Trimix_Enclosure_A2 (Autodesk Fusion 360 design; units mm, degrees)
description: designed concept
description: Owner measured 116.8x69.3x13.7; casing retained, factory back removed; interior drawing-derived
description: Drawing-derived visual reconstruction; connector positions and factory mounting holes require confirmation
description: nominal generic hardware; not supplier-authenticated CAD
part number: GEN-M3-BHCS-L8-AF2
part number: GEN-M3-HEATSET-OD4.2-L5
description: Owner-measured occupied FMA FPML1S2P050C envelope 42 W x 80.4 H x 20.35 D mm; pocket and local frame details provisional
description: Owner capacity 3400 mAh; 18.2 mm diameter x 69 mm cylinder is a dimensional visual reference, not measured cell CAD
description: RCY/BEC-style red two-wire battery disconnect retained by owner; provisional 12 x 10 x 4 mm reference body, not selected manufacturer CAD
description: RCY/BEC-style red disconnect mating reference; provisional 12 x 10 x 2.2 mm, not selected manufacturer CAD
description: 2 mm printed carrier; future PCB and disconnect notches, procurement pending
description: Space allocation only; no claim that the charging and sensor circuitry is routed or fitted
part number: GEN-M2-SHCS-L7-AF1.5
part number: GEN-M2-HEATSET-OD3.2-L4
description: Rear-release concept. Factory frame capture lip, pad contact and preload require measurement; not a validated display fastening detail
part number: GEN-M2-SHCS-L5-AF1.5
description: 12 mm purchased button; barrel, nut and terminals are conservative unmeasured references
description: Designed metal faceplate reference: 2.3 mm bulk, locally 1.80 mm; material/process and sealing unqualified; not a printed-wall exception
description: Designed removable printed support with >=2 mm nominal flange and boss walls; housing retention and physical fit unqualified
description: Provisional 13.6 x 16 x 0.60 mm board; connector straddle relief and mounting references only; no final circuit layout
description: GCT USB4720 Rev B drawing-derived reconstruction; manufacturer STEP download blocked. Simplified shell, tongue and gasket; not exact supplier CAD.
part number: USB4720-03-A-DRAWING-REFERENCE
description: GCT USB4720 Rev B drawing-derived reconstruction; manufacturer STEP download blocked. Simplified shell, tongue and gasket; not exact supplier CAD. Gasket is an uncompressed visual clearance reference, not seal simulation.
description: Illustrative contact stripes; not electrical pin geometry or PCB footprint
part number: GEN-M2-SHCS-L4-AF1.5
part number: GEN-M2-SHCS-L6-AF1.5
description: Designed printed L-clamp; 2 mm strap/stalk, 0.2 mm lateral stop clearance; physical fit and hand access pending
description: Separate 2 mm internal lid; gasket and seal groove deferred
description: Datasheet dimensional envelope: body Ø29.3x31.75, neck Ø16x6.5; no exact threads or supplier CAD
description: Unmeasured 6.5x10x10 connector and wire clearance
description: Drawing-derived PCB thickness1.6, can Ø20x16.7, opposite3.45 mm header allowance. Header profile and finishes illustrative; original total envelope remains reserved.
description: Full19x9.5x14 body rotated to X9.5,Y14,Z19; no manufacturer CAD available
description: Conservative clearance block for full26±1 mm leads, +Y orientation; not a physical solid lead bundle
description: Provisional12x17x5 GYBMEP envelope retained. Board thickness, pad holes, cap, IC placement and finishes are illustrative; module identity and all mounting dimensions remain unverified.
description: Nominal8 mm OD/5 mm ID straight fitting reference; actual part, flange, seal and hose bend unmeasured
description: Nominal4.4 mm OD feedthrough reference; wire potting, actual gland, cable diameter and bends unverified
description: Designed concept; nominal 2 mm walls; seal geometry and pressure qualification deferred
Autodesk Fusion 360 part; units mm, degrees
(part 1 of 6)
ref_plane "WorkPlane1" through (0, 0, 0) normal (0, 0, 1) x (1, 0, 0) in component "01 Tapered printed housing"
sketch "Front silhouette" plane through (0, 0, 0) normal (0, 0, 1) x (1, 0, 0) in component "01 Tapered printed housing"
  line L0 (0, 0) -> (75, 0)
  line L1 (75, 0) -> (75, 125)
  line L2 (75, 125) -> (0, 125)
  line L3 (0, 125) -> (0, 0)
  dimension "d45" = 75
  dimension "d46" = 125
  constraint horizontal L0
  constraint vertical L1
  constraint horizontal L2
  constraint vertical L3
  measures "d45" horizontal distance of L0.start L0.end
  measures "d46" vertical distance of L0.end L1.end
ref_plane "WorkPlane2" through (0, 0, 53.6) normal (0, 0, 1) x (1, 0, 0) in component "01 Tapered printed housing"
sketch "Rear silhouette" plane through (0, 0, 53.6) normal (0, 0, 1) x (1, 0, 0) in component "01 Tapered printed housing"
  line L0 (0.25, 0.25) -> (74.75, 0.25)
  line L1 (74.75, 0.25) -> (74.75, 124.75)
  line L2 (74.75, 124.75) -> (0.25, 124.75)
  line L3 (0.25, 124.75) -> (0.25, 0.25)
  dimension "d49" = 0.25
  dimension "d50" = 0.25
  dimension "d51" = 74.5
  dimension "d52" = 124.5
  constraint horizontal L0
  constraint vertical L1
  constraint horizontal L2
  constraint vertical L3
  measures "d49" horizontal distance of origin L0.start
  measures "d50" vertical distance of origin L0.start
  measures "d51" horizontal distance of L0.start L0.end
  measures "d52" vertical distance of L0.end L1.end
loft "Gentle rearward taper" add profiles "Front silhouette", "Rear silhouette" section 1 section 2 makes body 1 in component "01 Tapered printed housing"
fillet "Soft housing corners" radius 6 4 edges at (0.125, 0.125, 26.8) (0.125, 124.875, 26.8) (74.875, 0.125, 26.8) (74.875, 124.875, 26.8) on bodies 1 in component "01 Tapered printed housing"
ref_plane "WorkPlane3" through (0, 0, 14.5) normal (0, 0, 1) x (1, 0, 0) in component "01 Tapered printed housing"
sketch "Rear service cavity sketch" plane through (0, 0, 14.5) normal (0, 0, 1) x (1, 0, 0) in component "01 Tapered printed housing"
  line L0 (2.4, 2.4) -> (72.6, 2.4)
  line L1 (72.6, 2.4) -> (72.6, 122.6)
  line L2 (72.6, 122.6) -> (2.4, 122.6)
  line L3 (2.4, 122.6) -> (2.4, 2.4)
  dimension "d57" = 2.4
  dimension "d58" = 2.4
  dimension "d59" = 70.2
  dimension "d60" = 120.2
  constraint horizontal L0
  constraint vertical L1
  constraint horizontal L2
  constraint vertical L3
  measures "d57" horizontal distance of origin L0.start
  measures "d58" vertical distance of origin L0.start
  measures "d59" horizontal distance of L0.start L0.end
  measures "d60" vertical distance of L0.end L1.end
extrude "Rear service cavity" cut sketch "Rear service cavity sketch" along normal blind 56 bodies 1 in component "01 Tapered printed housing"
fillet "Inside cavity corner rounds" radius 3.6 4 edges at (72.6, 2.4, 34.05) (2.4, 2.4, 34.05) (2.4, 122.6, 34.05) (72.6, 122.6, 34.05) on bodies 1 in component "01 Tapered printed housing"
ref_plane "WorkPlane4" through (0, 0, -1) normal (0, 0, 1) x (1, 0, 0) in component "01 Tapered printed housing"
sketch "Front-removable factory display opening sketch" plane through (0, 0, -1) normal (0, 0, 1) x (1, 0, 0) in component "01 Tapered printed housing"
  line L0 (2.45, 3.7) -> (72.55, 3.7)
  line L1 (72.55, 3.7) -> (72.55, 121.3)
  line L2 (72.55, 121.3) -> (2.45, 121.3)
  line L3 (2.45, 121.3) -> (2.45, 3.7)
  dimension "d67" = 2.45
  dimension "d68" = 3.7
  dimension "d69" = 70.1
  dimension "d70" = 117.6
  constraint horizontal L0
  constraint vertical L1
  constraint horizontal L2
  constraint vertical L3
  measures "d67" horizontal distance of origin L0.start
  measures "d68" vertical distance of origin L0.start
  measures "d69" horizontal distance of L0.start L0.end
  measures "d70" vertical distance of L0.end L1.end
extrude "Front-removable factory display opening" cut sketch "Front-removable factory display opening sketch" along normal blind 16 bodies 1 in component "01 Tapered printed housing"
ref_plane "WorkPlane5" through (-1, 0, 0) normal (1, 0, 0) x (0, 1, 0) in component "01 Tapered printed housing"
sketch "Gas fitting wall passages sketch" plane through (-1, 0, 0) normal (1, 0, 0) x (0, 0, -1) in component "01 Tapered printed housing"
  circle A0 centre (-23, 105) radius 4.5
  dimension "d76" = 105
  dimension "d77" = 4.5
  measures "d76" vertical distance of origin A0.centre
  measures "d77" radius of A0
extrude "Gas fitting wall passages" cut sketch "Gas fitting wall passages sketch" along normal blind 77 bodies 1 in component "01 Tapered printed housing"
ref_plane "WorkPlane6" through (-1, 0, 0) normal (1, 0, 0) x (0, 1, 0) in component "01 Tapered printed housing"
sketch "Right button panel opening sketch" plane through (-1, 0, 0) normal (1, 0, 0) x (0, 0, -1) in component "01 Tapered printed housing"
  circle A0 centre (-44.5, 45) radius 6
  dimension "d83" = 45
  dimension "d84" = 6
  measures "d83" vertical distance of origin A0.centre
  measures "d84" radius of A0
extrude "Right button panel opening" cut sketch "Right button panel opening sketch" along normal blind 4.4 bodies 1 in component "01 Tapered printed housing"
ref_plane "WorkPlane7" through (71.6, 0, 0) normal (1, 0, 0) x (0, 1, 0) in component "01 Tapered printed housing"
sketch "Left USB insert opening sketch" plane through (71.6, 0, 0) normal (1, 0, 0) x (0, 0, -1) in component "01 Tapered printed housing"
  line L0 (-35, 6) -> (-19, 6)
  line L1 (-19, 6) -> (-19, 26)
  line L2 (-19, 26) -> (-35, 26)
  line L3 (-35, 26) -> (-35, 6)
  dimension "d89" = 35
  dimension "d90" = 6
  dimension "d91" = 16
  dimension "d92" = 20
  constraint horizontal L0
  constraint vertical L1
  constraint horizontal L2
  constraint vertical L3
  measures "d89" horizontal distance of origin L0.start
  measures "d90" vertical distance of origin L0.start
  measures "d91" horizontal distance of L0.start L0.end
  measures "d92" vertical distance of L0.end L1.end
extrude "Left USB insert opening" cut sketch "Left USB insert opening sketch" along normal blind 4.4 bodies 1 in component "01 Tapered printed housing"
ref_plane "WorkPlane1" through (0, 0, 53.8) normal (0, 0, 1) x (1, 0, 0) in component "02 Single rear cover"
sketch "Single screw-fastened rear cover sketch" plane through (0, 0, 53.8) normal (0, 0, 1) x (1, 0, 0) in component "02 Single rear cover"
  line L0 (0.25, 0.25) -> (74.75, 0.25)
  line L1 (74.75, 0.25) -> (74.75, 124.75)
  line L2 (74.75, 124.75) -> (0.25, 124.75)
  line L3 (0.25, 124.75) -> (0.25, 0.25)
  dimension "d97" = 0.25
  dimension "d98" = 0.25
  dimension "d99" = 74.5
  dimension "d100" = 124.5
  constraint horizontal L0
  constraint vertical L1
  constraint horizontal L2
  constraint vertical L3
  measures "d97" horizontal distance of origin L0.start
  measures "d98" vertical distance of origin L0.start
  measures "d99" horizontal distance of L0.start L0.end
  measures "d100" vertical distance of L0.end L1.end
extrude "Single screw-fastened rear cover" add sketch "Single screw-fastened rear cover sketch" along normal blind 2.2 separate body makes body 2 in component "02 Single rear cover"
fillet "Rear cover corner rounds" radius 6 4 edges at (0.25, 124.75, 54.9) (74.75, 124.75, 54.9) (74.75, 0.25, 54.9) (0.25, 0.25, 54.9) on bodies 2 in component "02 Single rear cover"
ref_plane "WorkPlane1" through (0, 0, 0.4) normal (0, 0, 1) x (1, 0, 0) in component "03 Guition factory casing — measured envelope"
sketch "Guition retained factory frame sketch" plane through (0, 0, 0.4) normal (0, 0, 1) x (1, 0, 0) in component "03 Guition factory casing — measured envelope"
  line L0 (2.85, 4.1) -> (72.15, 4.1)
  line L1 (72.15, 4.1) -> (72.15, 120.9)
  line L2 (72.15, 120.9) -> (2.85, 120.9)
  line L3 (2.85, 120.9) -> (2.85, 4.1)
  dimension "d107" = 2.85
  dimension "d108" = 4.1
  dimension "d109" = 69.3
  dimension "d110" = 116.8
  constraint horizontal L0
  constraint vertical L1
  constraint horizontal L2
  constraint vertical L3
  measures "d107" horizontal distance of origin L0.start
  measures "d108" vertical distance of origin L0.start
  measures "d109" horizontal distance of L0.start L0.end
  measures "d110" vertical distance of L0.end L1.end
extrude "Guition retained factory frame" add sketch "Guition retained factory frame sketch" along normal blind 13.7 separate body makes body 3 in component "03 Guition factory casing — measured envelope"
fillet "Factory frame corner reference" radius 2 4 edges at (2.85, 120.9, 7.25) (72.15, 120.9, 7.25) (72.15, 4.1, 7.25) (2.85, 4.1, 7.25) on bodies 3 in component "03 Guition factory casing — measured envelope"
ref_plane "WorkPlane2" through (0, 0, 3.4) normal (0, 0, 1) x (1, 0, 0) in component "03 Guition factory casing — measured envelope"
sketch "Factory open rear cavity sketch" plane through (0, 0, 3.4) normal (0, 0, 1) x (1, 0, 0) in component "03 Guition factory casing — measured envelope"
  line L0 (4.8, 8.5) -> (70.2, 8.5)
  line L1 (70.2, 8.5) -> (70.2, 116.5)
  line L2 (70.2, 116.5) -> (4.8, 116.5)
  line L3 (4.8, 116.5) -> (4.8, 8.5)
  dimension "d117" = 4.8
  dimension "d118" = 8.5
  dimension "d119" = 65.4
  dimension "d120" = 108
  constraint horizontal L0
  constraint vertical L1
  constraint horizontal L2
  constraint vertical L3
  measures "d117" horizontal distance of origin L0.start
  measures "d118" vertical distance of origin L0.start
  measures "d119" horizontal distance of L0.start L0.end
  measures "d120" vertical distance of L0.end L1.end
extrude "Factory open rear cavity" cut sketch "Factory open rear cavity sketch" along normal blind 12 bodies 3 in component "03 Guition factory casing — measured envelope"
ref_plane "WorkPlane3" through (0, 0, 0.3) normal (0, 0, 1) x (1, 0, 0) in component "03 Guition factory casing — measured envelope"
sketch "Factory glass recess sketch" plane through (0, 0, 0.3) normal (0, 0, 1) x (1, 0, 0) in component "03 Guition factory casing — measured envelope"
  line L0 (4.1, 5.3) -> (70.9, 5.3)
  line L1 (70.9, 5.3) -> (70.9, 119.7)
  line L2 (70.9, 119.7) -> (4.1, 119.7)
  line L3 (4.1, 119.7) -> (4.1, 5.3)
  dimension "d125" = 4.1
  dimension "d126" = 5.3
  dimension "d127" = 66.8
  dimension "d128" = 114.4
  constraint horizontal L0
  constraint vertical L1
  constraint horizontal L2
  constraint vertical L3
  measures "d125" horizontal distance of origin L0.start
  measures "d126" vertical distance of origin L0.start
  measures "d127" horizontal distance of L0.start L0.end
  measures "d128" vertical distance of L0.end L1.end
extrude "Factory glass recess" cut sketch "Factory glass recess sketch" along normal blind 1.3 bodies 3 in component "03 Guition factory casing — measured envelope"
ref_plane "WorkPlane1" through (0, 0, 0.4) normal (0, 0, 1) x (1, 0, 0) in component "04 Guition front glass — drawing reference"
sketch "Black border glass sketch" plane through (0, 0, 0.4) normal (0, 0, 1) x (1, 0, 0) in component "04 Guition front glass — drawing reference"
  line L0 (4.1, 5.3) -> (70.9, 5.3)
  line L1 (70.9, 5.3) -> (70.9, 119.7)
  line L2 (70.9, 119.7) -> (4.1, 119.7)
  line L3 (4.1, 119.7) -> (4.1, 5.3)
  dimension "d133" = 4.1
  dimension "d134" = 5.3
  dimension "d135" = 66.8
  dimension "d136" = 114.4
  constraint horizontal L0
  constraint vertical L1
  constraint horizontal L2
  constraint vertical L3
  measures "d133" horizontal distance of origin L0.start
  measures "d134" vertical distance of origin L0.start
  measures "d135" horizontal distance of L0.start L0.end
  measures "d136" vertical distance of L0.end L1.end
extrude "Black border glass" add sketch "Black border glass sketch" along normal blind 1.2 separate body makes body 4 in component "04 Guition front glass — drawing reference"
ref_plane "WorkPlane2" through (0, 0, 0.3) normal (0, 0, 1) x (1, 0, 0) in component "04 Guition front glass — drawing reference"
sketch "Active face recess sketch" plane through (0, 0, 0.3) normal (0, 0, 1) x (1, 0, 0) in component "04 Guition front glass — drawing reference"
  line L0 (9.42, 15.7) -> (65.58, 15.7)
  line L1 (65.58, 15.7) -> (65.58, 109.3)
  line L2 (65.58, 109.3) -> (9.42, 109.3)
  line L3 (9.42, 109.3) -> (9.42, 15.7)
  dimension "d141" = 9.42
  dimension "d142" = 15.7
  dimension "d143" = 56.16
  dimension "d144" = 93.6
  constraint horizontal L0
  constraint vertical L1
  constraint horizontal L2
  constraint vertical L3
  measures "d141" horizontal distance of origin L0.start
  measures "d142" vertical distance of origin L0.start
  measures "d143" horizontal distance of L0.start L0.end
  measures "d144" vertical distance of L0.end L1.end
extrude "Active face recess" cut sketch "Active face recess sketch" along normal blind 0.2 bodies 4 in component "04 Guition front glass — drawing reference"
ref_plane "WorkPlane1" through (0, 0, 0.4) normal (0, 0, 1) x (1, 0, 0) in component "05 Active 4.3 inch screen"
sketch "480x800 active area sketch" plane through (0, 0, 0.4) normal (0, 0, 1) x (1, 0, 0) in component "05 Active 4.3 inch screen"
  line L0 (9.42, 15.7) -> (65.58, 15.7)
  line L1 (65.58, 15.7) -> (65.58, 109.3)
  line L2 (65.58, 109.3) -> (9.42, 109.3)
  line L3 (9.42, 109.3) -> (9.42, 15.7)
  dimension "d149" = 9.42
  dimension "d150" = 15.7
  dimension "d151" = 56.16
  dimension "d152" = 93.6
  constraint horizontal L0
  constraint vertical L1
  constraint horizontal L2
  constraint vertical L3
  measures "d149" horizontal distance of origin L0.start
  measures "d150" vertical distance of origin L0.start
  measures "d151" horizontal distance of L0.start L0.end
  measures "d152" vertical distance of L0.end L1.end
extrude "480x800 active area" add sketch "480x800 active area sketch" along normal blind 0.1 separate body makes body 5 in component "05 Active 4.3 inch screen"
ref_plane "WorkPlane1" through (0, 0, 8) normal (0, 0, 1) x (1, 0, 0) in component "06 Guition PCB and connectors — illustrative detail"
sketch "Guition PCB outline reference sketch" plane through (0, 0, 8) normal (0, 0, 1) x (1, 0, 0) in component "06 Guition PCB and connectors — illustrative detail"
  line L0 (4.97, 8.5) -> (70.03, 8.5)
  line L1 (70.03, 8.5) -> (70.03, 116.5)
  line L2 (70.03, 116.5) -> (4.97, 116.5)
  line L3 (4.97, 116.5) -> (4.97, 8.5)
  dimension "d157" = 4.97
  dimension "d158" = 8.5
  dimension "d159" = 65.06
  dimension "d160" = 108
  constraint horizontal L0
  constraint vertical L1
  constraint horizontal L2
  constraint vertical L3
  measures "d157" horizontal distance of origin L0.start
  measures "d158" vertical distance of origin L0.start
  measures "d159" horizontal distance of L0.start L0.end
  measures "d160" vertical distance of L0.end L1.end
extrude "Guition PCB outline reference" add sketch "Guition PCB outline reference sketch" along normal blind 1.6 separate body makes body 6 in component "06 Guition PCB and connectors — illustrative detail"
ref_plane "WorkPlane2" through (0, 0, 7.9) normal (0, 0, 1) x (1, 0, 0) in component "06 Guition PCB and connectors — illustrative detail"
sketch "Factory mounting clearance reference sketch" plane through (0, 0, 7.9) normal (0, 0, 1) x (1, 0, 0) in component "06 Guition PCB and connectors — illustrative detail"
  circle A0 centre (7.5, 11.2) radius 2.5
  dimension "d165" = 7.5
  dimension "d166" = 11.2
  dimension "d167" = 2.5
  measures "d165" horizontal distance of origin A0.centre
  measures "d166" vertical distance of origin A0.centre
  measures "d167" radius of A0
extrude "Factory mounting clearance reference" cut sketch "Factory mounting clearance reference sketch" along normal blind 1.8 bodies 6 in component "06 Guition PCB and connectors — illustrative detail"
ref_plane "WorkPlane3" through (0, 0, 7.9) normal (0, 0, 1) x (1, 0, 0) in component "06 Guition PCB and connectors — illustrative detail"
sketch "Factory mounting clearance reference sketch (1)" plane through (0, 0, 7.9) normal (0, 0, 1) x (1, 0, 0) in component "06 Guition PCB and connectors — illustrative detail"
  circle A0 centre (7.5, 113.8) radius 2.5
  dimension "d172" = 7.5
  dimension "d173" = 113.8
  dimension "d174" = 2.5
  measures "d172" horizontal distance of origin A0.centre
  measures "d173" vertical distance of origin A0.centre
  measures "d174" radius of A0
extrude "Factory mounting clearance reference (1)" cut sketch "Factory mounting clearance reference sketch (1)" along normal blind 1.8 bodies 6 in component "06 Guition PCB and connectors — illustrative detail"
ref_plane "WorkPlane4" through (0, 0, 7.9) normal (0, 0, 1) x (1, 0, 0) in component "06 Guition PCB and connectors — illustrative detail"
sketch "Factory mounting clearance reference sketch (2)" plane through (0, 0, 7.9) normal (0, 0, 1) x (1, 0, 0) in component "06 Guition PCB and connectors — illustrative detail"
  circle A0 centre (67.5, 11.2) radius 2.5
  dimension "d179" = 67.5
  dimension "d180" = 11.2
  dimension "d181" = 2.5
  measures "d179" horizontal distance of origin A0.centre
  measures "d180" vertical distance of origin A0.centre
  measures "d181" radius of A0
extrude "Factory mounting clearance reference (2)" cut sketch "Factory mounting clearance reference sketch (2)" along normal blind 1.8 bodies 6 in component "06 Guition PCB and connectors — illustrative detail"
ref_plane "WorkPlane5" through (0, 0, 7.9) normal (0, 0, 1) x (1, 0, 0) in component "06 Guition PCB and connectors — illustrative detail"
sketch "Factory mounting clearance reference sketch (3)" plane through (0, 0, 7.9) normal (0, 0, 1) x (1, 0, 0) in component "06 Guition PCB and connectors — illustrative detail"
  circle A0 centre (67.5, 113.8) radius 2.5
  dimension "d186" = 67.5
  dimension "d187" = 113.8
  dimension "d188" = 2.5
  measures "d186" horizontal distance of origin A0.centre
  measures "d187" vertical distance of origin A0.centre
  measures "d188" radius of A0
extrude "Factory mounting clearance reference (3)" cut sketch "Factory mounting clearance reference sketch (3)" along normal blind 1.8 bodies 6 in component "06 Guition PCB and connectors — illustrative detail"
ref_plane "WorkPlane6" through (0, 0, 9.6) normal (0, 0, 1) x (1, 0, 0) in component "06 Guition PCB and connectors — illustrative detail"
sketch "ESP32-P4 visual reference sketch" plane through (0, 0, 9.6) normal (0, 0, 1) x (1, 0, 0) in component "06 Guition PCB and connectors — illustrative detail"
  line L0 (15, 75) -> (31, 75)
  line L1 (31, 75) -> (31, 91)
  line L2 (31, 91) -> (15, 91)
  line L3 (15, 91) -> (15, 75)
  dimension "d193" = 15
  dimension "d194" = 75
  dimension "d195" = 16
  dimension "d196" = 16
  constraint horizontal L0
  constraint vertical L1
  constraint horizontal L2
  constraint vertical L3
  measures "d193" horizontal distance of origin L0.start
  measures "d194" vertical distance of origin L0.start
  measures "d195" horizontal distance of L0.start L0.end
  measures "d196" vertical distance of L0.end L1.end
extrude "ESP32-P4 visual reference" add sketch "ESP32-P4 visual reference sketch" along normal blind 3 separate body makes body 7 in component "06 Guition PCB and connectors — illustrative detail"
ref_plane "WorkPlane7" through (0, 0, 9.6) normal (0, 0, 1) x (1, 0, 0) in component "06 Guition PCB and connectors — illustrative detail"
sketch "ESP32-C6 radio module reference sketch" plane through (0, 0, 9.6) normal (0, 0, 1) x (1, 0, 0) in component "06 Guition PCB and connectors — illustrative detail"
  line L0 (47, 90) -> (61, 90)
  line L1 (61, 90) -> (61, 109)
  line L2 (61, 109) -> (47, 109)
  line L3 (47, 109) -> (47, 90)
  dimension "d201" = 47
  dimension "d202" = 90
  dimension "d203" = 14
  dimension "d204" = 19
  constraint horizontal L0
  constraint vertical L1
  constraint horizontal L2
  constraint vertical L3
  measures "d201" horizontal distance of origin L0.start
  measures "d202" vertical distance of origin L0.start
  measures "d203" horizontal distance of L0.start L0.end
  measures "d204" vertical distance of L0.end L1.end
extrude "ESP32-C6 radio module reference" add sketch "ESP32-C6 radio module reference sketch" along normal blind 2.8 separate body makes body 8 in component "06 Guition PCB and connectors — illustrative detail"
ref_plane "WorkPlane8" through (0, 0, 9.6) normal (0, 0, 1) x (1, 0, 0) in component "06 Guition PCB and connectors — illustrative detail"
sketch "Memory package reference sketch" plane through (0, 0, 9.6) normal (0, 0, 1) x (1, 0, 0) in component "06 Guition PCB and connectors — illustrative detail"
  line L0 (34, 79) -> (41, 79)
  line L1 (41, 79) -> (41, 88)
  line L2 (41, 88) -> (34, 88)
  line L3 (34, 88) -> (34, 79)
  dimension "d209" = 34
  dimension "d210" = 79
  dimension "d211" = 7
  dimension "d212" = 9
  constraint horizontal L0
  constraint vertical L1
  constraint horizontal L2
  constraint vertical L3
  measures "d209" horizontal distance of origin L0.start
  measures "d210" vertical distance of origin L0.start
  measures "d211" horizontal distance of L0.start L0.end
  measures "d212" vertical distance of L0.end L1.end
extrude "Memory package reference" add sketch "Memory package reference sketch" along normal blind 1.2 separate body makes body 9 in component "06 Guition PCB and connectors — illustrative detail"
ref_plane "WorkPlane9" through (0, 0, 9.6) normal (0, 0, 1) x (1, 0, 0) in component "06 Guition PCB and connectors — illustrative detail"
sketch "Power inductor reference sketch" plane through (0, 0, 9.6) normal (0, 0, 1) x (1, 0, 0) in component "06 Guition PCB and connectors — illustrative detail"
  line L0 (14, 18) -> (20, 18)
  line L1 (20, 18) -> (20, 24)
  line L2 (20, 24) -> (14, 24)
  line L3 (14, 24) -> (14, 18)
  dimension "d217" = 14
  dimension "d218" = 18
  dimension "d219" = 6
  dimension "d220" = 6
  constraint horizontal L0
  constraint vertical L1
  constraint horizontal L2
  constraint vertical L3
  measures "d217" horizontal distance of origin L0.start
  measures "d218" vertical distance of origin L0.start
  measures "d219" horizontal distance of L0.start L0.end
  measures "d220" vertical distance of L0.end L1.end
extrude "Power inductor reference" add sketch "Power inductor reference sketch" along normal blind 3.4 separate body makes body 10 in component "06 Guition PCB and connectors — illustrative detail"
ref_plane "WorkPlane10" through (0, 0, 9.6) normal (0, 0, 1) x (1, 0, 0) in component "06 Guition PCB and connectors — illustrative detail"
sketch "Board IC reference sketch" plane through (0, 0, 9.6) normal (0, 0, 1) x (1, 0, 0) in component "06 Guition PCB and connectors — illustrative detail"
  line L0 (24, 23) -> (29, 23)
  line L1 (29, 23) -> (29, 28)
  line L2 (29, 28) -> (24, 28)
  line L3 (24, 28) -> (24, 23)
  dimension "d225" = 24
  dimension "d226" = 23
  dimension "d227" = 5
  dimension "d228" = 5
  constraint horizontal L0
  constraint vertical L1
  constraint horizontal L2
  constraint vertical L3
  measures "d225" horizontal distance of origin L0.start
  measures "d226" vertical distance of origin L0.start
  measures "d227" horizontal distance of L0.start L0.end
  measures "d228" vertical distance of L0.end L1.end
extrude "Board IC reference" add sketch "Board IC reference sketch" along normal blind 1.5 separate body makes body 11 in component "06 Guition PCB and connectors — illustrative detail"
ref_plane "WorkPlane11" through (0, 0, 9.6) normal (0, 0, 1) x (1, 0, 0) in component "06 Guition PCB and connectors — illustrative detail"
sketch "Rear USB connector reference sketch" plane through (0, 0, 9.6) normal (0, 0, 1) x (1, 0, 0) in component "06 Guition PCB and connectors — illustrative detail"
  line L0 (30, 9) -> (39, 9)
  line L1 (39, 9) -> (39, 16)
  line L2 (39, 16) -> (30, 16)
  line L3 (30, 16) -> (30, 9)
  dimension "d233" = 30
  dimension "d234" = 9
  dimension "d235" = 9
  dimension "d236" = 7
  constraint horizontal L0
  constraint vertical L1
  constraint horizontal L2
  constraint vertical L3
  measures "d233" horizontal distance of origin L0.start
  measures "d234" vertical distance of origin L0.start
  measures "d235" horizontal distance of L0.start L0.end
  measures "d236" vertical distance of L0.end L1.end
extrude "Rear USB connector reference" add sketch "Rear USB connector reference sketch" along normal blind 3.8 separate body makes body 12 in component "06 Guition PCB and connectors — illustrative detail"
ref_plane "WorkPlane12" through (0, 0, 9.6) normal (0, 0, 1) x (1, 0, 0) in component "06 Guition PCB and connectors — illustrative detail"
sketch "Display FPC latch reference sketch" plane through (0, 0, 9.6) normal (0, 0, 1) x (1, 0, 0) in component "06 Guition PCB and connectors — illustrative detail"
  line L0 (23, 62) -> (51, 62)
  line L1 (51, 62) -> (51, 66)
  line L2 (51, 66) -> (23, 66)
  line L3 (23, 66) -> (23, 62)
  dimension "d241" = 23
  dimension "d242" = 62
  dimension "d243" = 28
  dimension "d244" = 4
  constraint horizontal L0
  constraint vertical L1
  constraint horizontal L2
  constraint vertical L3
  measures "d241" horizontal distance of origin L0.start
  measures "d242" vertical distance of origin L0.start
  measures "d243" horizontal distance of L0.start L0.end
  measures "d244" vertical distance of L0.end L1.end
extrude "Display FPC latch reference" add sketch "Display FPC latch reference sketch" along normal blind 1.8 separate body makes body 13 in component "06 Guition PCB and connectors — illustrative detail"
ref_plane "WorkPlane13" through (0, 0, 9.6) normal (0, 0, 1) x (1, 0, 0) in component "06 Guition PCB and connectors — illustrative detail"
sketch "Expansion header reference sketch" plane through (0, 0, 9.6) normal (0, 0, 1) x (1, 0, 0) in component "06 Guition PCB and connectors — illustrative detail"
  line L0 (52, 34) -> (57, 34)
  line L1 (57, 34) -> (57, 67)
  line L2 (57, 67) -> (52, 67)
  line L3 (52, 67) -> (52, 34)
  dimension "d249" = 52
  dimension "d250" = 34
  dimension "d251" = 5
  dimension "d252" = 33
  constraint horizontal L0
  constraint vertical L1
  constraint horizontal L2
  constraint vertical L3
  measures "d249" horizontal distance of origin L0.start
  measures "d250" vertical distance of origin L0.start
  measures "d251" horizontal distance of L0.start L0.end
  measures "d252" vertical distance of L0.end L1.end
extrude "Expansion header reference" add sketch "Expansion header reference sketch" along normal blind 4 separate body makes body 14 in component "06 Guition PCB and connectors — illustrative detail"
fillet "Radiused forward display aperture preserves corner walls" radius 2.4 4 edges at (72.55, 3.7, 7.5) (72.55, 121.3, 7.5) (2.45, 3.7, 7.5) (2.45, 121.3, 7.5) on bodies 1 in component "01 Tapered printed housing"
ref_plane "WorkPlane8" through (0, 0, 43) normal (0, 0, 1) x (1, 0, 0) in component "01 Tapered printed housing"
sketch "Rear M3 boss sketch" plane through (0, 0, 43) normal (0, 0, 1) x (1, 0, 0) in component "01 Tapered printed housing"
  circle A0 centre (6, 6) radius 4.2
  dimension "d259" = 6
  dimension "d260" = 6
  dimension "d261" = 4.2
  measures "d259" horizontal distance of origin A0.centre
  measures "d260" vertical distance of origin A0.centre
  measures "d261" radius of A0
extrude "Rear M3 boss" add sketch "Rear M3 boss sketch" along normal blind 8.6 bodies 1 in component "01 Tapered printed housing"
ref_plane "WorkPlane9" through (0, 0, 46.15) normal (0, 0, 1) x (1, 0, 0) in component "01 Tapered printed housing"
sketch "Sketch9" plane through (0, 0, 46.15) normal (0, 0, 1) x (1, 0, 0) in component "01 Tapered printed housing"
  circle A0 centre (6, 6) radius 2.15
  dimension "d266" = 6
  dimension "d267" = 6
  dimension "d268" = 2.15
  measures "d266" horizontal distance of origin A0.centre
  measures "d267" vertical distance of origin A0.centre
  measures "d268" radius of A0
extrude "M3 insert pocket — supplier fit TBD" cut sketch "Sketch9" along normal blind 5.55 bodies 1 in component "01 Tapered printed housing"
ref_plane "WorkPlane2" through (0, 0, 52.35) normal (0, 0, 1) x (1, 0, 0) in component "02 Single rear cover"
sketch "Local 2 mm screw bearing pad sketch" plane through (0, 0, 52.35) normal (0, 0, 1) x (1, 0, 0) in component "02 Single rear cover"
  circle A0 centre (6, 6) radius 5.2
  dimension "d273" = 6
  dimension "d274" = 6
  dimension "d275" = 5.2
  measures "d273" horizontal distance of origin A0.centre
  measures "d274" vertical distance of origin A0.centre
  measures "d275" radius of A0
ref_plane "WorkPlane3" through (0, 0, 52.25) normal (0, 0, 1) x (1, 0, 0) in component "02 Single rear cover"
sketch "Rear M3 through clearance sketch" plane through (0, 0, 52.25) normal (0, 0, 1) x (1, 0, 0) in component "02 Single rear cover"
  circle A0 centre (6, 6) radius 1.7
  dimension "d280" = 6
  dimension "d281" = 6
  dimension "d282" = 1.7
  measures "d280" horizontal distance of origin A0.centre
  measures "d281" vertical distance of origin A0.centre
  measures "d282" radius of A0
extrude "Rear M3 through clearance" cut sketch "Rear M3 through clearance sketch" along normal blind 4 bodies 2 in component "02 Single rear cover"
ref_plane "WorkPlane4" through (0, 0, 54.35) normal (0, 0, 1) x (1, 0, 0) in component "02 Single rear cover"
sketch "Recessed M3 button head sketch" plane through (0, 0, 54.35) normal (0, 0, 1) x (1, 0, 0) in component "02 Single rear cover"
  circle A0 centre (6, 6) radius 3.05
  dimension "d287" = 6
  dimension "d288" = 6
  dimension "d289" = 3.05
  measures "d287" horizontal distance of origin A0.centre
  measures "d288" vertical distance of origin A0.centre
  measures "d289" radius of A0
ref_plane "WorkPlane10" through (0, 0, 43) normal (0, 0, 1) x (1, 0, 0) in component "01 Tapered printed housing"
sketch "Rear M3 boss sketch (1)" plane through (0, 0, 43) normal (0, 0, 1) x (1, 0, 0) in component "01 Tapered printed housing"
  circle A0 centre (69, 6) radius 4.2
  dimension "d294" = 69
  dimension "d295" = 6
  dimension "d296" = 4.2
  measures "d294" horizontal distance of origin A0.centre
  measures "d295" vertical distance of origin A0.centre
  measures "d296" radius of A0
extrude "Rear M3 boss (1)" add sketch "Rear M3 boss sketch (1)" along normal blind 8.6 bodies 1 in component "01 Tapered printed housing"
ref_plane "WorkPlane11" through (0, 0, 46.15) normal (0, 0, 1) x (1, 0, 0) in component "01 Tapered printed housing"
sketch "Sketch11" plane through (0, 0, 46.15) normal (0, 0, 1) x (1, 0, 0) in component "01 Tapered printed housing"
  circle A0 centre (69, 6) radius 2.15
  dimension "d301" = 69
  dimension "d302" = 6
  dimension "d303" = 2.15
  measures "d301" horizontal distance of origin A0.centre
  measures "d302" vertical distance of origin A0.centre
  measures "d303" radius of A0
extrude "M3 insert pocket — supplier fit TBD (1)" cut sketch "Sketch11" along normal blind 5.55 bodies 1 in component "01 Tapered printed housing"
ref_plane "WorkPlane5" through (0, 0, 52.35) normal (0, 0, 1) x (1, 0, 0) in component "02 Single rear cover"
sketch "Local 2 mm screw bearing pad sketch (1)" plane through (0, 0, 52.35) normal (0, 0, 1) x (1, 0, 0) in component "02 Single rear cover"
  circle A0 centre (69, 6) radius 5.2
  dimension "d308" = 69
  dimension "d309" = 6
  dimension "d310" = 5.2
  measures "d308" horizontal distance of origin A0.centre
  measures "d309" vertical distance of origin A0.centre
  measures "d310" radius of A0
ref_plane "WorkPlane6" through (0, 0, 52.25) normal (0, 0, 1) x (1, 0, 0) in component "02 Single rear cover"
sketch "Rear M3 through clearance sketch (1)" plane through (0, 0, 52.25) normal (0, 0, 1) x (1, 0, 0) in component "02 Single rear cover"
  circle A0 centre (69, 6) radius 1.7
  dimension "d315" = 69
  dimension "d316" = 6
  dimension "d317" = 1.7
  measures "d315" horizontal distance of origin A0.centre
  measures "d316" vertical distance of origin A0.centre
  measures "d317" radius of A0
extrude "Rear M3 through clearance (1)" cut sketch "Rear M3 through clearance sketch (1)" along normal blind 4 bodies 2 in component "02 Single rear cover"
ref_plane "WorkPlane7" through (0, 0, 54.35) normal (0, 0, 1) x (1, 0, 0) in component "02 Single rear cover"
sketch "Recessed M3 button head sketch (1)" plane through (0, 0, 54.35) normal (0, 0, 1) x (1, 0, 0) in component "02 Single rear cover"
  circle A0 centre (69, 6) radius 3.05
  dimension "d322" = 69
  dimension "d323" = 6
  dimension "d324" = 3.05
  measures "d322" horizontal distance of origin A0.centre
  measures "d323" vertical distance of origin A0.centre
  measures "d324" radius of A0
ref_plane "WorkPlane12" through (0, 0, 43) normal (0, 0, 1) x (1, 0, 0) in component "01 Tapered printed housing"
sketch "Rear M3 boss sketch (2)" plane through (0, 0, 43) normal (0, 0, 1) x (1, 0, 0) in component "01 Tapered printed housing"
  circle A0 centre (6, 119) radius 4.2
  dimension "d329" = 6
  dimension "d330" = 119
  dimension "d331" = 4.2
  measures "d329" horizontal distance of origin A0.centre
  measures "d330" vertical distance of origin A0.centre
  measures "d331" radius of A0
extrude "Rear M3 boss (2)" add sketch "Rear M3 boss sketch (2)" along normal blind 8.6 bodies 1 in component "01 Tapered printed housing"
ref_plane "WorkPlane13" through (0, 0, 46.15) normal (0, 0, 1) x (1, 0, 0) in component "01 Tapered printed housing"
sketch "Sketch13" plane through (0, 0, 46.15) normal (0, 0, 1) x (1, 0, 0) in component "01 Tapered printed housing"
  circle A0 centre (6, 119) radius 2.15
  dimension "d336" = 6
  dimension "d337" = 119
  dimension "d338" = 2.15
  measures "d336" horizontal distance of origin A0.centre
  measures "d337" vertical distance of origin A0.centre
  measures "d338" radius of A0
extrude "M3 insert pocket — supplier fit TBD (2)" cut sketch "Sketch13" along normal blind 5.55 bodies 1 in component "01 Tapered printed housing"
ref_plane "WorkPlane8" through (0, 0, 52.35) normal (0, 0, 1) x (1, 0, 0) in component "02 Single rear cover"
sketch "Local 2 mm screw bearing pad sketch (2)" plane through (0, 0, 52.35) normal (0, 0, 1) x (1, 0, 0) in component "02 Single rear cover"
  circle A0 centre (6, 119) radius 5.2
  dimension "d343" = 6
  dimension "d344" = 119
  dimension "d345" = 5.2
  measures "d343" horizontal distance of origin A0.centre
  measures "d344" vertical distance of origin A0.centre
  measures "d345" radius of A0
ref_plane "WorkPlane9" through (0, 0, 52.25) normal (0, 0, 1) x (1, 0, 0) in component "02 Single rear cover"
sketch "Rear M3 through clearance sketch (2)" plane through (0, 0, 52.25) normal (0, 0, 1) x (1, 0, 0) in component "02 Single rear cover"
  circle A0 centre (6, 119) radius 1.7
  dimension "d350" = 6
  dimension "d351" = 119
  dimension "d352" = 1.7
  measures "d350" horizontal distance of origin A0.centre
  measures "d351" vertical distance of origin A0.centre
  measures "d352" radius of A0
extrude "Rear M3 through clearance (2)" cut sketch "Rear M3 through clearance sketch (2)" along normal blind 4 bodies 2 in component "02 Single rear cover"
ref_plane "WorkPlane10" through (0, 0, 54.35) normal (0, 0, 1) x (1, 0, 0) in component "02 Single rear cover"
sketch "Recessed M3 button head sketch (2)" plane through (0, 0, 54.35) normal (0, 0, 1) x (1, 0, 0) in component "02 Single rear cover"
  circle A0 centre (6, 119) radius 3.05
  dimension "d357" = 6
  dimension "d358" = 119
  dimension "d359" = 3.05
  measures "d357" horizontal distance of origin A0.centre
  measures "d358" vertical distance of origin A0.centre
  measures "d359" radius of A0
ref_plane "WorkPlane14" through (0, 0, 43) normal (0, 0, 1) x (1, 0, 0) in component "01 Tapered printed housing"
sketch "Rear M3 boss sketch (3)" plane through (0, 0, 43) normal (0, 0, 1) x (1, 0, 0) in component "01 Tapered printed housing"
  circle A0 centre (69, 119) radius 4.2
  dimension "d364" = 69
  dimension "d365" = 119
  dimension "d366" = 4.2
  measures "d364" horizontal distance of origin A0.centre
  measures "d365" vertical distance of origin A0.centre
  measures "d366" radius of A0
extrude "Rear M3 boss (3)" add sketch "Rear M3 boss sketch (3)" along normal blind 8.6 bodies 1 in component "01 Tapered printed housing"
ref_plane "WorkPlane15" through (0, 0, 46.15) normal (0, 0, 1) x (1, 0, 0) in component "01 Tapered printed housing"
sketch "Sketch15" plane through (0, 0, 46.15) normal (0, 0, 1) x (1, 0, 0) in component "01 Tapered printed housing"
  circle A0 centre (69, 119) radius 2.15
  dimension "d371" = 69
  dimension "d372" = 119
  dimension "d373" = 2.15
  measures "d371" horizontal distance of origin A0.centre
  measures "d372" vertical distance of origin A0.centre
  measures "d373" radius of A0
extrude "M3 insert pocket — supplier fit TBD (3)" cut sketch "Sketch15" along normal blind 5.55 bodies 1 in component "01 Tapered printed housing"
ref_plane "WorkPlane11" through (0, 0, 52.35) normal (0, 0, 1) x (1, 0, 0) in component "02 Single rear cover"
sketch "Local 2 mm screw bearing pad sketch (3)" plane through (0, 0, 52.35) normal (0, 0, 1) x (1, 0, 0) in component "02 Single rear cover"
  circle A0 centre (69, 119) radius 5.2
  dimension "d378" = 69
  dimension "d379" = 119
  dimension "d380" = 5.2
  measures "d378" horizontal distance of origin A0.centre
  measures "d379" vertical distance of origin A0.centre
  measures "d380" radius of A0
ref_plane "WorkPlane12" through (0, 0, 52.25) normal (0, 0, 1) x (1, 0, 0) in component "02 Single rear cover"
sketch "Rear M3 through clearance sketch (3)" plane through (0, 0, 52.25) normal (0, 0, 1) x (1, 0, 0) in component "02 Single rear cover"
  circle A0 centre (69, 119) radius 1.7
  dimension "d385" = 69
  dimension "d386" = 119
  dimension "d387" = 1.7
  measures "d385" horizontal distance of origin A0.centre
  measures "d386" vertical distance of origin A0.centre
  measures "d387" radius of A0
extrude "Rear M3 through clearance (3)" cut sketch "Rear M3 through clearance sketch (3)" along normal blind 4 bodies 2 in component "02 Single rear cover"
ref_plane "WorkPlane13" through (0, 0, 54.35) normal (0, 0, 1) x (1, 0, 0) in component "02 Single rear cover"
sketch "Recessed M3 button head sketch (3)" plane through (0, 0, 54.35) normal (0, 0, 1) x (1, 0, 0) in component "02 Single rear cover"
  circle A0 centre (69, 119) radius 3.05
  dimension "d392" = 69
  dimension "d393" = 119
  dimension "d394" = 3.05
  measures "d392" horizontal distance of origin A0.centre
  measures "d393" vertical distance of origin A0.centre
  measures "d394" radius of A0
ref_plane "WorkPlane1" through (0, 0, -8) normal (0, 0, 1) x (1, 0, 0) in component "M3 x 8 button screw — GEN-M3-BHCS-L8-AF2"
sketch "Joined screw sketch" plane through (0, 0, -8) normal (0, 0, 1) x (1, 0, 0) in component "M3 x 8 button screw — GEN-M3-BHCS-L8-AF2"
  circle A0 centre (0, 0) radius 1.45
  dimension "d399" = 1.45
  measures "d399" radius of A0
extrude "Joined screw" add sketch "Joined screw sketch" along normal blind 8 separate body makes body 15 in component "M3 x 8 button screw — GEN-M3-BHCS-L8-AF2"
ref_plane "WorkPlane2" through (0, 0, 0) normal (0, 0, 1) x (1, 0, 0) in component "M3 x 8 button screw — GEN-M3-BHCS-L8-AF2"
sketch "Screw head sketch" plane through (0, 0, 0) normal (0, 0, 1) x (1, 0, 0) in component "M3 x 8 button screw — GEN-M3-BHCS-L8-AF2"
  circle A0 centre (0, 0) radius 2.85
  dimension "d404" = 2.85
  measures "d404" radius of A0
extrude "Screw head" add sketch "Screw head sketch" along normal blind 1.65 bodies 15 in component "M3 x 8 button screw — GEN-M3-BHCS-L8-AF2"
fillet "Rounded head crown" radius 0.95 1 edges at (-2.6571, -1.0306, 1.65) on bodies 15 in component "M3 x 8 button screw — GEN-M3-BHCS-L8-AF2"
ref_plane "WorkPlane3" through (0, 0, 0.65) normal (0, 0, 1) x (1, 0, 0) in component "M3 x 8 button screw — GEN-M3-BHCS-L8-AF2"
sketch "Hex drive 2 mm across flats" plane through (0, 0, 0.65) normal (0, 0, 1) x (1, 0, 0) in component "M3 x 8 button screw — GEN-M3-BHCS-L8-AF2"
  line L0 (1.1547, 0) -> (0.5774, 1)
  line L1 (0.5774, 1) -> (-0.5774, 1)
  line L2 (-0.5774, 1) -> (-1.1547, 0)
  line L3 (-1.1547, 0) -> (-0.5774, -1)
  line L4 (-0.5774, -1) -> (0.5774, -1)
  line L5 (0.5774, -1) -> (1.1547, 0)
extrude "Hex drive recess" cut sketch "Hex drive 2 mm across flats" along normal blind 1.1 bodies 15 in component "M3 x 8 button screw — GEN-M3-BHCS-L8-AF2"
ref_plane "WorkPlane1" through (0, 0, -5) normal (0, 0, 1) x (1, 0, 0) in component "M3 insert OD4.2 x 5 — GEN-M3-HEATSET-OD4.2-L5"
sketch "Hollow insert sketch" plane through (0, 0, -5) normal (0, 0, 1) x (1, 0, 0) in component "M3 insert OD4.2 x 5 — GEN-M3-HEATSET-OD4.2-L5"
  circle A0 centre (0, 0) radius 2.1
  dimension "d415" = 2.1
  measures "d415" radius of A0
extrude "Hollow insert" add sketch "Hollow insert sketch" along normal blind 5 separate body makes body 16 in component "M3 insert OD4.2 x 5 — GEN-M3-HEATSET-OD4.2-L5"
ref_plane "WorkPlane2" through (0, 0, -5.1) normal (0, 0, 1) x (1, 0, 0) in component "M3 insert OD4.2 x 5 — GEN-M3-HEATSET-OD4.2-L5"
sketch "Unthreaded insert bore sketch" plane through (0, 0, -5.1) normal (0, 0, 1) x (1, 0, 0) in component "M3 insert OD4.2 x 5 — GEN-M3-HEATSET-OD4.2-L5"
  circle A0 centre (0, 0) radius 1.55
  dimension "d420" = 1.55
  measures "d420" radius of A0
extrude "Unthreaded insert bore" cut sketch "Unthreaded insert bore sketch" along normal blind 5.2 bodies 16 in component "M3 insert OD4.2 x 5 — GEN-M3-HEATSET-OD4.2-L5"
ref_plane "WorkPlane3" through (0, 0, -3.75) normal (0, 0, 1) x (1, 0, 0) in component "M3 insert OD4.2 x 5 — GEN-M3-HEATSET-OD4.2-L5"
sketch "Cosmetic insert relief" plane through (0, 0, -3.75) normal (0, 0, 1) x (1, 0, 0) in component "M3 insert OD4.2 x 5 — GEN-M3-HEATSET-OD4.2-L5"
  circle A0 centre (0, 0) radius 2.2
  circle A1 centre (0, 0) radius 2
  dimension "d425" = 2.2
  dimension "d426" = 2
  measures "d425" radius of A0
  measures "d426" radius of A1
extrude "Cosmetic annular relief" cut sketch "Cosmetic insert relief" along normal blind 0.25 bodies 16 in component "M3 insert OD4.2 x 5 — GEN-M3-HEATSET-OD4.2-L5"
ref_plane "WorkPlane4" through (0, 0, -1.25) normal (0, 0, 1) x (1, 0, 0) in component "M3 insert OD4.2 x 5 — GEN-M3-HEATSET-OD4.2-L5"
sketch "Cosmetic insert relief (1)" plane through (0, 0, -1.25) normal (0, 0, 1) x (1, 0, 0) in component "M3 insert OD4.2 x 5 — GEN-M3-HEATSET-OD4.2-L5"
  circle A0 centre (0, 0) radius 2.2
  circle A1 centre (0, 0) radius 2
  dimension "d431" = 2.2
  dimension "d432" = 2
  measures "d431" radius of A0
  measures "d432" radius of A1
extrude "Cosmetic annular relief (1)" cut sketch "Cosmetic insert relief (1)" along normal blind 0.25 bodies 16 in component "M3 insert OD4.2 x 5 — GEN-M3-HEATSET-OD4.2-L5"
ref_plane "WorkPlane1" through (0, 0, 16.7) normal (0, 0, 1) x (1, 0, 0) in component "Battery / FMA protected holder - owner-measured envelope"
sketch "Measured occupied holder outer frame sketch" plane through (0, 0, 16.7) normal (0, 0, 1) x (1, 0, 0) in component "Battery / FMA protected holder - owner-measured envelope"
  line L0 (3, 4.2) -> (45, 4.2)
  line L1 (45, 4.2) -> (45, 84.6)
  line L2 (45, 84.6) -> (3, 84.6)
  line L3 (3, 84.6) -> (3, 4.2)
  dimension "d437" = 3
  dimension "d438" = 4.2
  dimension "d439" = 42
  dimension "d440" = 80.4
  constraint horizontal L0
  constraint vertical L1
  constraint horizontal L2
  constraint vertical L3
  measures "d437" horizontal distance of origin L0.start
  measures "d438" vertical distance of origin L0.start
  measures "d439" horizontal distance of L0.start L0.end
  measures "d440" vertical distance of L0.end L1.end
extrude "Measured occupied holder outer frame" add sketch "Measured occupied holder outer frame sketch" along normal blind 20.35 separate body makes body 17 in component "Battery / FMA protected holder - owner-measured envelope"
fillet "Provisional holder outer corner rounds" radius 1 4 edges at (3, 84.6, 26.875) (45, 84.6, 26.875) (45, 4.2, 26.875) (3, 4.2, 26.875) on bodies 17 in component "Battery / FMA protected holder - owner-measured envelope"
ref_plane "WorkPlane2" through (0, 0, 17.8) normal (0, 0, 1) x (1, 0, 0) in component "Battery / FMA protected holder - owner-measured envelope"
sketch "Open occupied cell pocket sketch" plane through (0, 0, 17.8) normal (0, 0, 1) x (1, 0, 0) in component "Battery / FMA protected holder - owner-measured envelope"
  line L0 (4, 6.2) -> (44, 6.2)
  line L1 (44, 6.2) -> (44, 82.6)
  line L2 (44, 82.6) -> (4, 82.6)
  line L3 (4, 82.6) -> (4, 6.2)
  dimension "d447" = 4
  dimension "d448" = 6.2
  dimension "d449" = 40
  dimension "d450" = 76.4
  constraint horizontal L0
  constraint vertical L1
  constraint horizontal L2
  constraint vertical L3
  measures "d447" horizontal distance of origin L0.start
  measures "d448" vertical distance of origin L0.start
  measures "d449" horizontal distance of L0.start L0.end
  measures "d450" vertical distance of L0.end L1.end
extrude "Open occupied cell pocket" cut sketch "Open occupied cell pocket sketch" along normal blind 20.35 bodies 17 in component "Battery / FMA protected holder - owner-measured envelope"
ref_plane "WorkPlane1" through (0, 9.2, 0) normal (0, 1, 0) x (0, 0, 1) in component "Battery / 18650 cell A - owner-rated 3400 mAh"
sketch "Cell axial cylinder sketch" plane through (0, 9.2, 0) normal (0, 1, 0) x (1, 0, 0) in component "Battery / 18650 cell A - owner-rated 3400 mAh"
  circle A0 centre (13.8, -26.95) radius 9.1
  dimension "d455" = 13.8
  dimension "d456" = 26.95
  dimension "d457" = 9.1
  measures "d455" horizontal distance of origin A0.centre
  measures "d456" vertical distance of origin A0.centre
  measures "d457" radius of A0
extrude "Blue 18650 reference cylinder" add sketch "Cell axial cylinder sketch" along normal blind 69 separate body makes body 18 in component "Battery / 18650 cell A - owner-rated 3400 mAh"
ref_plane "WorkPlane1" through (0, 9.2, 0) normal (0, 1, 0) x (0, 0, 1) in component "Battery / 18650 cell B - owner-rated 3400 mAh"